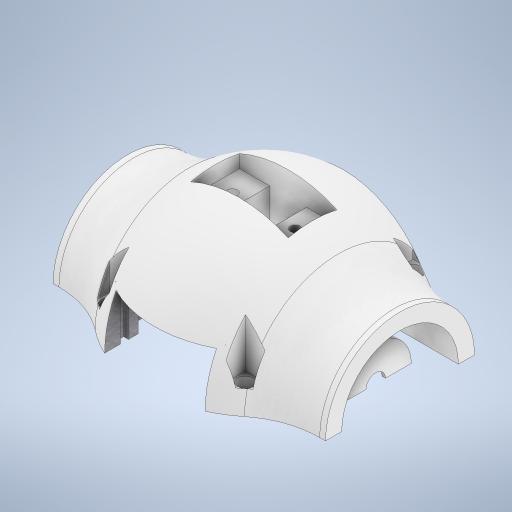
# Autodesk Inventor part: body front moter middle lemon shape
Saved by Autodesk Inventor 2023 (Build 270158000, 158)
## iProperties
Created: 2022-10-08
Part Number: body front moter middle lemon shape
Material: ABS プラスチック
Document SubType Name: Modeling
Designer: ellie
Density: 1.06 g/cm^3
Appearance: 積雪
Author: ellie
Autodesk Inventor part; units mm, degrees
sketch "スケッチ1" plane through (0, 0, 0) normal (0, 1, 0) x (-1, 0, 0)
  circle A0 centre (0, 0) radius 37
  line L0 (0, 0) -> (0, -37)
  line L1 (0, 0) -> (0, 37)
  dimension "d0" = 74
  constraints: 4 end point, 2 point on circle, 2 vertical, 1 centre point, 1 coincident
  measures "d0" diameter of A0
revolve "回転1" add sketch "スケッチ1" angle 180 about axis through (0, 0, 0) along (0, 0, 1) picked at (-2.7444, -24.3574) contours L1 L0 A0
sketch "スケッチ5" plane through (0, 0, 0) normal (0, -1, 0) x (1, 0, 0)
  line L0 (-21, -20.5) -> (21, -20.5)
  line L1 (21, -20.5) -> (21, -8.5)
  line L2 (21, -8.5) -> (-21, -8.5)
  line L3 (-21, -8.5) -> (-21, -20.5)
  line L4 (-21, -10.5) -> (-21, -8.5)
  line L5 (0, 28.75) -> (-17, 28.75)
  line L6 (-17, 28.75) -> (-17, 26.25)
  line L7 (-17, 26.25) -> (0, 26.25)
  line L8 (0, 26.25) -> (0, 28.75)
  line L9 (0, 23.25) -> (-20.5, 23.25)
  line L10 (-20.5, 23.25) -> (-20.5, 21.75)
  line L11 (-20.5, 21.75) -> (0, 21.75)
  line L12 (0, 21.75) -> (0, 23.25)
  line L13 (0, 15.75) -> (-21.5, 15.75)
  line L14 (-21.5, 15.75) -> (-21.5, 13.25)
  line L15 (-21.5, 13.25) -> (0, 13.25)
  line L16 (0, 13.25) -> (0, 15.75)
  line L17 (0, 7.25) -> (-24, 7.25)
  line L18 (-24, 7.25) -> (-24, 5.25)
  line L19 (-24, 5.25) -> (0, 5.25)
  line L20 (0, 5.25) -> (0, 7.25)
  circle A0 centre (0, 0) radius 37 projected
  circle A1 centre (0, 0) radius 37 projected
  line L21 (0, 37) -> (0, -37)
  line L22 (37, 0) -> (-37, 0)
  line L23 (-33.5, 5.25) -> (-24, 5.25)
  line L24 (-24, 5.25) -> (-24, -5.25)
  line L25 (-24, -5.25) -> (-33.5, -5.25)
  line L26 (-33.5, -5.25) -> (-33.5, 5.25)
  line L27 (-24, -8.0262) -> (-24, 5.25)
  line L28 (-29, 22.9783) -> (-29, -22.9783)
  line L29 (-15.5, 28.75) -> (0, 28.75)
  line L30 (0, 28.75) -> (0, 37)
  line L31 (0, 37) -> (-15.5, 37)
  line L32 (-15.5, 37) -> (-15.5, 28.75)
  line L33 (-15.5, 26.25) -> (0, 26.25)
  line L34 (0, 26.25) -> (0, 23.25)
  line L35 (0, 23.25) -> (-15.5, 23.25)
  line L36 (-15.5, 23.25) -> (-15.5, 26.25)
  line L37 (-19, 15.75) -> (0, 15.75)
  line L38 (0, 15.75) -> (0, 21.75)
  line L39 (0, 21.75) -> (-19, 21.75)
  line L40 (-19, 21.75) -> (-19, 15.75)
  line L41 (-19, 13.25) -> (0, 13.25)
  line L42 (0, 13.25) -> (0, 7.25)
  line L43 (0, 7.25) -> (-19, 7.25)
  line L44 (-19, 7.25) -> (-19, 13.25)
  line L45 (-24, 0) -> (-40.9365, 0)
  line L46 (-24, 0) -> (-9.0837, 0)
  line L47 (-9, 5.25) -> (-24, 5.25)
  line L48 (-24, 5.25) -> (-24, -5.25)
  line L49 (-24, -5.25) -> (-9, -5.25)
  line L50 (-9, 5.25) -> (-24, -5.25) construction
  line L51 (-24, 5.25) -> (-9, -5.25) construction
  line L52 (-24, 7.25) -> (-34.5, 7.25)
  line L53 (-34.5, 7.25) -> (-34.5, -7.25)
  line L54 (-34.5, -7.25) -> (-24, -7.25)
  line L55 (-24, -7.25) -> (-24, 7.25)
  line L56 (-24, 7.25) -> (-34.5, -7.25) construction
  line L57 (-34.5, 7.25) -> (-24, -7.25) construction
  line L58 (-8.35, 5.25) -> (-1, 5.25)
  line L59 (-1, 5.25) -> (-1, -5.25)
  line L60 (-1, -5.25) -> (-8.35, -5.25)
  line L61 (-8.35, 5.25) -> (-1, -5.25) construction
  line L62 (-1, 5.25) -> (-8.35, -5.25) construction
  line L63 (-24, 5.25) -> (-29, 5.25)
  line L64 (-24, -5.25) -> (-29, -5.25)
  line L65 (-24, 7.25) -> (-29, 7.25)
  line L66 (-24, -7.25) -> (-29, -7.25)
  line L67 (27.7263, -24.5) -> (-27.7263, -24.5)
  line L68 (-8.35, 5.25) -> (-6.8, 5.25)
  line L69 (-6.6281, -5.25) -> (-7.8281, -5.25)
  line L70 (0, 7.25) -> (1, 7.25)
  line L71 (0, -3) -> (0, 7.25)
  line L72 (-12.5791, -8.5) -> (-9, -8.5)
  point P0 (0, -20.5)
  point P1 (0, -8.5)
  point P2 (0, 27.5)
  point P3 (0, 22.5)
  point P4 (0, 14.5)
  point P5 (0, 6.25)
  point P6 (-21, -14.5)
  point P7 (-27, -0.5262)
  point P8 (-29, 22.9783)
  point P9 (-29, -22.9783)
  point P10 (-29, -5.25)
  point P11 (-15.5, 24.75)
  point P12 (-15.5, 33.5969)
  point P13 (0, 28.75)
  point P14 (0, 37)
  point P15 (0, 26.25)
  point P16 (0, 13.25)
  point P17 (0, 15.75)
  point P18 (-29, 0)
  point P19 (-33.5, 0)
  point P20 (-24, 0)
  point P21 (-16.5, 0)
  point P22 (-29.25, 0)
  point P23 (-4.675, 0)
  point P24 (-27, 0.5)
  point P25 (-28, 0.4738)
  point P26 (-28, -11.5262)
  point P27 (-27, -11.5)
  point P28 (-24, -5.25)
  point P29 (-24, -5.25)
  point P30 (-24, -5.25)
  point P31 (-24, 5.25)
  point P32 (-24, -5.25)
  point P33 (-1, 0)
  point P34 (-8, 5.25)
  point P35 (-27.7263, -24.5)
  point P36 (-8, -5.25)
  point P37 (0, 5.25)
  point P38 (-29, -7.25)
  point P39 (-29, 7.25)
  point P40 (-24, -1.3881)
  dimension "d12" = 42
  dimension "d13" = 12
  dimension "d23" = 17
  dimension "d24" = 2.5
  dimension "d27" = 20.5
  dimension "d28" = 1.5
  dimension "d30" = 21.5
  dimension "d31" = 2.5
  dimension "d33" = 2
  dimension "d88" = 0
  dimension "d89" = 0
  dimension "d90" = 16.5
  dimension "d92" = 21
  dimension "d97" = 9.5
  dimension "d98" = 10.5
  dimension "d113" = 29
  dimension "d122" = 15.5
  dimension "d124" = 3
  dimension "d125" = 15.5
  dimension "d126" = 6
  dimension "d127" = 6
  dimension "d161" = 14.5
  dimension "d162" = 10.5
  dimension "d164" = 10.5
  dimension "d170" = 24.5
  dimension "d187" = 1
  dimension "d283" = 23
  dimension "d284" = 10.5
  dimension "d285" = 15
  dimension "d286" = 34.5
  dimension "d287" = 1
  dimension "d288" = 19
  dimension "d289" = 19
  constraints: 144 end point, 26 parallel, 19 horizontal, 16 midpoint, 16 perpendicular, 15 point on line, 9 collinear, 1 vertical, 20 other
  measures "d12" distance of L2.end L1.end
  measures "d13" distance of L1.end L0.end
  measures "d23" distance of L7.end L6.end
  measures "d24" distance of L6.end L5.end
  measures "d27" distance of L11.end L10.end
  measures "d28" distance of L10.end L9.end
  measures "d30" distance of L15.end L14.end
  measures "d31" distance of L14.end L13.end
  measures "d33" distance of L18.end L17.end
  measures "d89" distance from line of point (0, 0) L22
  measures "d90" distance from line of L0 point (0, -37)
  measures "d92" distance of the line from the sketch origin of L3
  measures "d97" distance of L24.end L25.end
  measures "d98" distance of L23.end L24.end
  measures "d113" distance of the line from the sketch origin of L28
  measures "d122" distance of the line from the sketch origin of L32
  measures "d124" distance of L33.end L34.end
  measures "d126" distance of L38.end L37.end
  measures "d127" distance of L41.end L42.end
  measures "d161" distance between parallel lines of L54 L52
  measures "d162" distance between parallel lines of L48 L53
  measures "d164" distance between parallel lines of L60 L58
  measures "d170" distance between parallel lines of L67 L22
  measures "d187" distance between parallel lines of L71 L59
  measures "d283" distance between parallel lines of L55 L59
  measures "d284" distance between parallel lines of L49 L47
  measures "d285" distance of L48.end L49.end
  measures "d286" distance of the line from the sketch origin of L53
  measures "d287" distance of the line from the sketch origin of L59
  measures "d288" distance of the line from the sketch origin of L40
  measures "d289" distance of the line from the sketch origin of L44
extrude "GNSボード" cut sketch "スケッチ5" against normal blind 16 contours L8 L7 L6 L5
extrude "GNSボード止めるよう" cut sketch "スケッチ5" against normal blind 15 contours L21 L5 L32 A0 | L21 L9 L36 L7
extrude "アルミ板１" cut sketch "スケッチ5" against normal blind 20 contours L12 L11 L10 L9
extrude "メイン基板" cut sketch "スケッチ5" against normal blind 21 contours L15 L14 L13 L16
extrude "メイン止めるよう" cut sketch "スケッチ5" against normal blind 16.5 contours L17 L44 L15 L21 | L13 L40 L11 L21
extrude "アルミ板２" cut sketch "スケッチ5" against normal blind 20 contours L19 L18 L17 L20
extrude "電池ボックス入れ" cut sketch "スケッチ5" against normal blind 13 contours L3 L2 L21 L0 | L21 L2 L1 L0
extrude "side ut" cut sketch "スケッチ5" against normal blind 100 contours A0 L22 L53 L54 L28 | A0 L28 L52 L53 L22 | L54 L53 L22 L26 L25 L28 | L53 L52 L28 L23 L26 L22 | L25 L26 L22 L28 | L26 L23 L28 L22
extrude "motor case" add sketch "スケッチ5" against normal blind 7 contours L54 L53 L22 L26 L25 L28 | L28 L25 L27 L54 | L53 L52 L28 L23 L26 L22 | L28 L22 L24 L25 | L25 L26 L22 L28 | L22 L28 L23 L24 | L52 L18 L23 L28 | L26 L23 L28 L22
extrude "bottom cut" cut sketch "スケッチ5" against normal blind 90 contours L67 A0 L21 | L21 A0 L67
extrude "motor" cut sketch "スケッチ5" against normal blind 6 contours L28 L22 L24 L25 | L25 L26 L22 L28 | L22 L28 L23 L24 | L26 L23 L28 L22
extrude "motor block" [suppressed]
sketch "スケッチ26" plane through (-34.5, 0, -7.25) normal (-1, 0, 0) x (0, 0, 1)
  line L0 (14.5, 0) -> (0, 0) projected
  circle A0 centre (7.25, 0) radius 3
  point P0 (7.25, 0)
  point P1 (7.25, 0)
  point P2 (4.25, 0)
  point P3 (10.25, 0)
  dimension "d197" = 6
  constraints: 1 centre point, 1 coincident
  measures "d197" diameter of A0
extrude "押し出し34" cut sketch "スケッチ26" against normal blind 27 contours L0 A0 picked at (7.9985, 0.6631)
mirror "ミラー11" about plane through (0, 0, 0) normal (1, 0, 0) of "GNSボード", "GNSボード止めるよう", "アルミ板１", "メイン止めるよう", "メイン基板", "アルミ板２", "motor", "押し出し34", "motor case", "電池ボックス入れ", "side ut"
ref_plane "作業平面5" through (0, 13, 0) normal (0, -1, 0) x (1, 0, 0)
ref_plane "作業平面6" through (-15.5, 37, 28.75) normal (0, -1, 0) x (1, 0, 0)
sketch "スケッチ29" plane through (-15.5, 37, 28.75) normal (0, -1, 0) x (1, 0, 0)
  line L0 (15.5, -28.75) -> (-67.7134, -28.75)
  line L1 (-67.7134, -28.75) -> (15.5, -28.75)
  line L2 (110.7852, -24.5555) -> (110.7852, -27.3413)
  line L3 (15.5, -28.75) -> (98.1975, -28.75)
  circle A0 centre (25.2, -28.75) radius 1.5
  circle A1 centre (5.8, -28.75) radius 1.5
  line L4 (32.4245, 0) -> (-1.4245, 0) projected
  line L5 (15.5, 0) -> (15.5, -53.25)
  line L6 (-12.2263, -53.25) -> (43.2263, -53.25) projected
  point P0 (32.5, 0)
  point P1 (-1.5, 0)
  point P2 (43.2263, -53.25)
  point P3 (-11.5, -52)
  point P4 (42.5, -52)
  dimension "d205" = 3
  dimension "d206" = 19.4
  dimension "d207" = 0
  constraints: 10 end point, 2 centre point, 2 horizontal, 1 collinear, 1 midpoint, 1 vertical, 3 other
  measures "d205" diameter of A0
  measures "d206" distance of A1.centre A0.centre
  measures "d207" distance from line of L3 A0.centre
extrude "押し出し36" cut sketch "スケッチ29" along normal blind 25
sketch "スケッチ30" plane through (-15.5, 37, 28.75) normal (0, -1, 0) x (1, 0, 0)
  line L0 (0.5, -21.25) -> (30.5, -21.25)
  line L1 (30.5, -21.25) -> (30.5, -36.25)
  line L2 (30.5, -36.25) -> (0.5, -36.25)
  line L3 (0.5, -36.25) -> (0.5, -21.25)
  line L4 (0.5, -21.25) -> (30.5, -36.25) construction
  line L5 (30.5, -21.25) -> (0.5, -36.25) construction
  point P0 (15.5, -28.75)
  dimension "d210" = 30
  dimension "d211" = 15
  constraints: 12 end point, 2 midpoint, 2 parallel, 1 horizontal, 1 perpendicular
  measures "d210" distance of L1.end L2.end
  measures "d211" distance of L0.end L1.end
extrude "押し出し37" cut sketch "スケッチ30" along normal blind 8
ref_plane "作業平面7" through (-15.5, 12, 28.75) normal (0, 1, 0) x (1, 0, 0)
sketch "スケッチ33" plane through (-15.5, 12, 28.75) normal (0, 1, 0) x (1, 0, 0)
  circle A0 centre (25.2, 28.75) radius 1.5 projected
  circle A1 centre (5.8, 28.75) radius 1.5 projected
  line L0 (0.5, 36.25) -> (0.5, 21.25) projected
  line L1 (30.5, 21.25) -> (30.5, 36.25) projected
  line L2 (0.5, 21.25) -> (30.5, 21.25) projected
  line L3 (30.5, 36.25) -> (0.5, 36.25) projected
  line L4 (15.5, 0) -> (15.5, 53.25) projected
  line L5 (15.5, 28.75) -> (98.1975, 28.75) projected
  circle A2 centre (25.2, 28.75) radius 3
  circle A3 centre (5.8, 28.75) radius 3
  dimension "d219" = 6
  dimension "d220" = 6
  constraints: 2 centre point, 2 coincident
  measures "d219" diameter of A2
  measures "d220" diameter of A3
extrude "押し出し39" cut sketch "スケッチ33" along normal blind 10 contours L5 A0 | L5 A2 A0 | A0 L5 A2 | A0 L5 | A1 | A3
sketch "スケッチ35" plane through (-17, 0, 26.25) normal (0, -1, 0) x (1, 0, 0)
  circle A0 centre (-4, 0.4) radius 2.4
  line L0 (-16.5, -21) -> (-7, -21) projected
  line L1 (-16.5, -31.5) -> (-16.5, -21) projected
  line L2 (-7, -31.5) -> (-16.5, -31.5) projected
  line L3 (-17.5, -23.25) -> (-16.5, -23.25) projected
  line L4 (-16.5, -23.25) -> (-16.5, -21) projected
  line L5 (-16.5, -21) -> (-7, -21) projected
  line L6 (-7, -21) -> (-7, -19) projected
  line L7 (-7, -19) -> (-2, -19) projected
  line L8 (-2, -19) -> (-2, -13) projected
  line L9 (-2, -13) -> (-4.5, -13) projected
  line L10 (-4.5, -13) -> (-4.5, -10.5) projected
  line L11 (-4.5, -10.5) -> (-2, -10.5) projected
  line L12 (-2, -10.5) -> (-2, -4.5) projected
  line L13 (-2, -4.5) -> (-3.5, -4.5) projected
  line L14 (-3.5, -4.5) -> (-3.5, -3) projected
  line L15 (-3.5, -3) -> (1.5, -3) projected
  line L16 (1.5, -3) -> (1.5, 0) projected
  line L17 (1.5, 0) -> (0, 0) projected
  line L18 (0, 0) -> (0, 2.5) projected
  line L19 (0, 2.5) -> (1.5, 2.5) projected
  line L20 (1.5, 2.5) -> (1.5, 7.3469) projected
  arc A1 (1.5, 7.3469) -> (-12, -3.2717) centre (17, -26.25) ccw projected
  line L21 (-12, -3.2717) -> (-12, -19) projected
  line L22 (-12, -19) -> (-17.5, -19) projected
  line L23 (-17.5, -19) -> (-17.5, -23.25) projected
  line L24 (-7, -21) -> (-7, -31.5) projected
  dimension "d231" = 4.8
  dimension "d233" = 1
  dimension "d234" = 4
  constraints: 1 centre point
  measures "d231" diameter of A0
  measures "d233" distance edge to line of A0 L15
  measures "d234" distance from line of A0.centre L18
extrude "押し出し41" cut sketch "スケッチ35" against normal blind 20 contours A0
mirror "ミラー12" about plane through (0, 0, 0) normal (1, 0, 0) of "押し出し41"
sketch "スケッチ36" plane through (-34.5, 0, -7.25) normal (0, -1, 0) x (1, 0, 0)
  circle A0 centre (9.5, -13.75) radius 2.4
  line L0 (58.5, 4.25) -> (42, 4.25) projected
  line L1 (58.5, 12.5) -> (10.5, 12.5) projected
  line L2 (27, 4.25) -> (10.5, 4.25) projected
  line L3 (10.5, 12.5) -> (10.5, 14.5) projected
  line L4 (1, 2) -> (1, 4.25) projected
  line L5 (1, 4.25) -> (0, 4.25) projected
  line L6 (0, 4.25) -> (0, 0) projected
  line L7 (0, 0) -> (5.5, 0) projected
  line L8 (5.5, 0) -> (5.5, -15.7283) projected
  arc A1 (5.5, -15.7283) -> (6.7737, -17.25) centre (34.5, 7.25) ccw projected
  line L9 (6.7737, -17.25) -> (62.2263, -17.25) projected
  arc A2 (62.2263, -17.25) -> (63.5, -15.7283) centre (34.5, 7.25) ccw projected
  line L10 (63.5, -15.7283) -> (63.5, 0) projected
  line L11 (69, 0) -> (63.5, 0) projected
  line L12 (69, 4.25) -> (69, 0) projected
  line L13 (69, 4.25) -> (68, 4.25) projected
  line L14 (68, 4.25) -> (68, 2) projected
  line L15 (58.5, 14.5) -> (58.5, 12.5) projected
  line L16 (13.5, -1.25) -> (55.5, -1.25) projected
  line L17 (55.5, -1.25) -> (55.5, -13.25) projected
  line L18 (55.5, -13.25) -> (13.5, -13.25) projected
  line L19 (13.5, -13.25) -> (13.5, -1.25) projected
  line L20 (55.5, -1.25) -> (55.5, -13.25) projected
  line L21 (13.5, -1.25) -> (55.5, -1.25) projected
  line L22 (13.5, -13.25) -> (13.5, -1.25) projected
  line L23 (55.5, -13.25) -> (13.5, -13.25) projected
  line L24 (0, 10.25) -> (1, 10.25) projected
  line L25 (1, 10.25) -> (1, 12.5) projected
  line L26 (1, 12.5) -> (10.5, 12.5) projected
  line L27 (10.5, 14.5) -> (15.5, 14.5) projected
  line L28 (15.5, 14.5) -> (15.5, 20.5) projected
  line L29 (15.5, 20.5) -> (13, 20.5) projected
  line L30 (13, 20.5) -> (13, 23) projected
  line L31 (13, 23) -> (15.5, 23) projected
  line L32 (15.5, 23) -> (15.5, 29) projected
  line L33 (15.5, 29) -> (14, 29) projected
  line L34 (14, 29) -> (14, 30.5) projected
  line L35 (14, 30.5) -> (19, 30.5) projected
  line L36 (19, 30.5) -> (19, 33.5) projected
  line L37 (19, 33.5) -> (17.5, 33.5) projected
  line L38 (17.5, 33.5) -> (17.5, 36) projected
  line L39 (17.5, 36) -> (19, 36) projected
  line L40 (19, 36) -> (19, 40.8469) projected
  line L41 (5.5, 30.2283) -> (5.5, 14.5) projected
  line L42 (5.5, 14.5) -> (0, 14.5) projected
  line L43 (0, 14.5) -> (0, 10.25) projected
  line L44 (10.5, 10.25) -> (27, 10.25) projected
  line L45 (10.5, 2) -> (1, 2) projected
  line L46 (68, 2) -> (58.5, 2) projected
  line L47 (42, 10.25) -> (58.5, 10.25) projected
  line L48 (68, 10.25) -> (69, 10.25) projected
  line L49 (69, 14.5) -> (69, 10.25) projected
  line L50 (63.5, 14.5) -> (69, 14.5) projected
  line L51 (63.5, 14.5) -> (63.5, 30.2283) projected
  line L52 (50, 40.8469) -> (50, 36) projected
  line L53 (50, 36) -> (51.5, 36) projected
  line L54 (51.5, 36) -> (51.5, 33.5) projected
  line L55 (51.5, 33.5) -> (50, 33.5) projected
  line L56 (50, 33.5) -> (50, 30.5) projected
  line L57 (50, 30.5) -> (55, 30.5) projected
  line L58 (55, 30.5) -> (55, 29) projected
  line L59 (55, 29) -> (53.5, 29) projected
  line L60 (53.5, 29) -> (53.5, 23) projected
  line L61 (53.5, 23) -> (56, 23) projected
  line L62 (56, 23) -> (56, 20.5) projected
  line L63 (56, 20.5) -> (53.5, 20.5) projected
  line L64 (53.5, 20.5) -> (53.5, 14.5) projected
  line L65 (53.5, 14.5) -> (58.5, 14.5) projected
  line L66 (58.5, 12.5) -> (68, 12.5) projected
  line L67 (68, 12.5) -> (68, 10.25) projected
  circle A3 centre (13.5, 33.9) radius 2.4 projected
  circle A4 centre (55.5, 33.9) radius 2.4 projected
  arc A5 (19, 40.8469) -> (5.5, 30.2283) centre (34.5, 7.25) ccw projected
  arc A6 (63.5, 30.2283) -> (50, 40.8469) centre (34.5, 7.25) ccw projected
  line L68 (58.5, 2) -> (58.5, 4.25) projected
  line L69 (42, 4.25) -> (42, 10.25) projected
  line L70 (58.5, 10.25) -> (58.5, 12.5) projected
  line L71 (10.5, 12.5) -> (10.5, 10.25) projected
  line L72 (27, 10.25) -> (27, 4.25) projected
  line L73 (10.5, 4.25) -> (10.5, 2) projected
  dimension "d237" = 4.8
  dimension "d238" = 4
  constraints: 1 centre point
  measures "d237" diameter of A0
  measures "d238" distance from line of A0.centre L19
extrude "押し出し42" cut sketch "スケッチ36" against normal blind 25 contours A0
mirror "ミラー13" about plane through (0, 0, 0) normal (1, 0, 0) of "押し出し42"
ref_plane "作業平面8" through (-17, 35, 26.25) normal (0, -1, 0) x (1, 0, 0)
sketch "スケッチ37" plane through (-17, 35, 26.25) normal (0, -1, 0) x (1, 0, 0)
  line L0 (38.5, -10.5) -> (-4.5, -10.5) projected
  line L1 (2, -18.75) -> (2, -33.75) projected
  line L2 (32, -33.75) -> (32, -18.75) projected
  arc A0 (32.5, 3.8124) -> (1.5, 3.8124) centre (17, -26.25) ccw projected
  line L3 (32.5, 3.8124) -> (32.5, 7.3469) projected
  line L4 (46, -3.2717) -> (46, -49.2283) projected
  arc A1 (44.7263, -50.75) -> (46, -49.2283) centre (17, -26.25) ccw projected
  line L5 (44.7263, -50.75) -> (-10.7263, -50.75) projected
  arc A2 (-12, -49.2283) -> (-10.7263, -50.75) centre (17, -26.25) ccw projected
  line L6 (-12, -49.2283) -> (-12, -3.2717) projected
  line L7 (1.5, 7.3469) -> (1.5, 3.8124) projected
  line L8 (-7, 3.4) -> (-1, 3.4)
  line L9 (-1, 3.4) -> (-1, -2.6)
  line L10 (-1, -2.6) -> (-7, -2.6)
  line L11 (-7, -2.6) -> (-7, 3.4)
  arc A3 (37.6, -40) -> (37.6, -40) centre (-4, 0.4) ccw projected
  line L12 (-7, 3.4) -> (-1, -2.6) construction
  line L13 (-1, 3.4) -> (-7, -2.6) construction
  line L14 (41, 3.4) -> (35, 3.4)
  line L15 (35, 3.4) -> (35, -2.6)
  line L16 (35, -2.6) -> (41, -2.6)
  line L17 (41, -2.6) -> (41, 3.4)
  arc A4 (37.6, -40) -> (37.6, -40) centre (38, 0.4) ccw projected
  line L18 (41, 3.4) -> (35, -2.6) construction
  line L19 (35, 3.4) -> (41, -2.6) construction
  line L20 (-5, -44.25) -> (-11, -44.25)
  line L21 (-11, -44.25) -> (-11, -50.25)
  line L22 (-11, -50.25) -> (-5, -50.25)
  line L23 (-5, -50.25) -> (-5, -44.25)
  circle A5 centre (-8, -47.25) radius 2.4 projected
  line L24 (-5, -44.25) -> (-11, -50.25) construction
  line L25 (-11, -44.25) -> (-5, -50.25) construction
  line L26 (45, -44.25) -> (39, -44.25)
  line L27 (39, -44.25) -> (39, -50.25)
  line L28 (39, -50.25) -> (45, -50.25)
  line L29 (45, -50.25) -> (45, -44.25)
  circle A6 centre (42, -47.25) radius 2.4 projected
  line L30 (45, -44.25) -> (39, -50.25) construction
  line L31 (39, -44.25) -> (45, -50.25) construction
  line L32 (32, -18.75) -> (2, -18.75) projected
  line L33 (2, -33.75) -> (32, -33.75) projected
  arc A7 (46, -3.2717) -> (32.5, 7.3469) centre (17, -26.25) ccw projected
  arc A8 (1.5, 7.3469) -> (-12, -3.2717) centre (17, -26.25) ccw projected
  point P0 (-3.6, -40)
  point P1 (36.5, 1.5)
  point P2 (-2.5, 1.5)
  dimension "d243" = 6
  dimension "d244" = 6
  dimension "d245" = 6
  dimension "d246" = 6
  dimension "d247" = 6
  dimension "d248" = 6
  dimension "d249" = 6
  dimension "d250" = 6
  constraints: 48 end point, 8 midpoint, 8 parallel, 4 horizontal, 4 perpendicular, 10 other
  measures "d243" distance of L9.end L10.end
  measures "d244" distance of L8.end L9.end
  measures "d245" distance of L16.end L15.end
  measures "d246" distance of L15.end L14.end
  measures "d247" distance of L22.end L21.end
  measures "d248" distance of L21.end L20.end
  measures "d249" distance of L28.end L27.end
  measures "d250" distance of L27.end L26.end
extrude "押し出し43" cut sketch "スケッチ37" along normal blind 20 contours L23 L22 L21 L20 | A5 | L29 L28 L27 L26 | A6
extrude "押し出し44" cut sketch "スケッチ37" along normal blind 28 contours A4 L8 L9 L10 | L10 L11 A8 L8 A4 | L11 L8 A8 | A7 L14 L17 | L17 L16 L15 L14 A7
sketch "スケッチ39" plane through (-15.5, 29, 28.75) normal (0, 1, 0) x (1, 0, 0)
  line L0 (21.2, 21.25) -> (9.8, 21.25)
  line L1 (9.8, 21.25) -> (9.8, 36.25)
  line L2 (9.8, 36.25) -> (21.2, 36.25)
  line L3 (21.2, 36.25) -> (21.2, 21.25)
  line L4 (21.2, 21.25) -> (9.8, 36.25) construction
  line L5 (9.8, 21.25) -> (21.2, 36.25) construction
  circle A0 centre (5.8, 28.75) radius 1.5 projected
  circle A1 centre (25.2, 28.75) radius 1.5 projected
  line L6 (0.5, 21.25) -> (30.5, 21.25) projected
  line L7 (30.5, 36.25) -> (0.5, 36.25) projected
  circle A2 centre (5.8, 28.75) radius 1.5 projected
  circle A3 centre (25.2, 28.75) radius 1.5 projected
  line L8 (0.5, 36.25) -> (30.5, 36.25) projected
  line L9 (0.5, 21.25) -> (0.5, 36.25) projected
  line L10 (30.5, 21.25) -> (0.5, 21.25) projected
  line L11 (30.5, 36.25) -> (30.5, 21.25) projected
  point P0 (15.5, 28.75)
  dimension "d255" = 4
  dimension "d256" = 0
  constraints: 12 end point, 2 midpoint, 2 parallel, 1 horizontal, 1 perpendicular
  measures "d255" distance from line of L1 A0.centre
  measures "d256" distance between parallel lines of L6 L0
extrude "押し出し45" cut sketch "スケッチ39" against normal up to surface (12.5 mm away) contours L0 L1 L2 L3
ref_plane "作業平面9" through (42, 0, -7.25) normal (1, 0, 0) x (0, 0, -1)
sketch "スケッチ41" plane through (42, 0, -7.25) normal (1, 0, 0) x (0, 0, -1)
  arc A0 (-4.25, 0) -> (-10.25, 0) centre (-7.25, 0) ccw projected
  arc A1 (-4.25, 0) -> (-10.25, 0) centre (-7.25, 0) ccw projected
  line L0 (-4.25, 0) -> (0, 0) projected
  line L1 (0, 0) -> (0, 7) projected
  line L2 (0, 7) -> (-14.5, 7) projected
  line L3 (-14.5, 0) -> (-14.5, 7) projected
  line L4 (-14.5, 0) -> (-10.25, 0) projected
  line L5 (0, 7) -> (0, 0) projected
  line L6 (15.7283, 0) -> (0, 0) projected
  arc A2 (15.7283, 0) -> (-30.2283, 0) centre (-7.25, 0) ccw projected
  line L7 (-14.5, 0) -> (-30.2283, 0) projected
  line L8 (-14.5, 0) -> (-14.5, 7) projected
  line L9 (-14.5, 7) -> (0, 7) projected
  line L10 (-2, 0) -> (-12, 0) projected
  line L11 (-2, 0) -> (-2, 6) projected
  line L12 (-12, 6) -> (-2, 6) projected
  line L13 (-12, 0) -> (-12, 6) projected
  circle A3 centre (-7.25, 0) radius 23
  circle A4 centre (-7.25, 0) radius 18
  point P0 (-25.25, 0)
  point P1 (10.75, 0)
  dimension "d267" = 46
  dimension "d268" = 36
  constraints: 2 centre point, 2 coincident
  measures "d267" diameter of A3
  measures "d268" diameter of A4
extrude "押し出し47" add sketch "スケッチ41" against normal up to surface (13 mm away) contours A4 L7 A2 L6
fillet "面フィレット1" radius 27.7 1 edges at (29, 22.9783, 0)
mirror "ミラー14" about plane through (0, 0, 0) normal (1, 0, 0) of "面フィレット1", "押し出し47"
sketch "スケッチ42" plane through (0, 16.5, 0) normal (0, -1, 0) x (1, 0, 0)
  line L0 (-5.7, 7.5) -> (5.7, 7.5) projected
  line L1 (-5.7, 5.25) -> (-5.7, 7.25) projected
  line L2 (5.7, 7.25) -> (5.7, 5.25) projected
  line L3 (15, 7.5) -> (5.7, 7.5) projected
  line L4 (5.7, 7.5) -> (-5.7, 7.5)
  line L5 (-5.7, 7.5) -> (-5.7, 10.5)
  line L6 (-5.7, 10.5) -> (5.7, 10.5)
  line L7 (5.7, 10.5) -> (5.7, 7.5)
  point P0 (0, 0)
  point P1 (-5.7, 7.5)
  dimension "d272" = 3
  constraints: 8 end point, 3 parallel, 1 horizontal, 1 perpendicular
  measures "d272" distance of L6.end L0.end
extrude "押し出し48" cut sketch "スケッチ42" against normal blind 10
sketch "スケッチ43" plane through (34.5, 0, -3) normal (1, 0, 0) x (0, 0, -1)
  arc A0 (0, 0) -> (-6, 0) centre (-3, 0) ccw projected
  circle A1 centre (-3, 0) radius 11
  arc A2 (15, 0) -> (-21, 0) centre (-3, 0) ccw projected
  line L0 (-10.25, 0) -> (-21, 0) projected
  line L1 (-10.25, 0) -> (-10.25, 7) projected
  line L2 (-10.25, 7) -> (4.25, 7) projected
  line L3 (4.25, 7) -> (4.25, 0) projected
  line L4 (15, 0) -> (4.25, 0) projected
  line L5 (-10.25, 0) -> (-6, 0) projected
  line L6 (0, 0) -> (4.25, 0) projected
  line L7 (2, 0) -> (-8, 0) projected
  point P0 (-3, 0)
  point P1 (8, 0)
  point P2 (-14, 0)
  dimension "d275" = 22
  constraints: 1 centre point, 1 coincident
  measures "d275" diameter of A1
extrude "押し出し49" add sketch "スケッチ43" against normal up to surface (5.5 mm away) contours L3 L2 L1 L0 A1 L4
mirror "ミラー15" about plane through (0, 0, 0) normal (1, 0, 0) of "押し出し49"
sketch "スケッチ44" plane through (-34.5, 0, 0) normal (-1, 0, 0) x (0, 0, 1)
  point P0 (0, 0)
sketch "スケッチ45" plane through (-29, 0, 0) normal (-1, 0, 0) x (0, 0, 1)
  circle A0 centre (0, 0) radius 11
  arc A1 (3, 0) -> (-3, 0) centre (0, 0) ccw projected
  circle A2 centre (0, 0) radius 18
  line L0 (18, 0) -> (11, 0) projected
  line L1 (-11, 0) -> (-18, 0) projected
  point P0 (0, 0)
  dimension "d278" = 22
  dimension "d279" = 36
  constraints: 2 centre point, 2 coincident
  measures "d278" diameter of A0
  measures "d279" diameter of A2
extrude "押し出し50" cut sketch "スケッチ45" against normal blind 5 contours A0 L1 A2 L0 picked at (-15.4923, 1.4359)
mirror "ミラー16" about plane through (0, 0, 0) normal (1, 0, 0) of "押し出し50"
